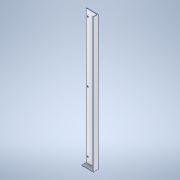
# Autodesk Inventor part: Guias de bandeja 1
Saved by Autodesk Inventor 2020 (Build 240168000, 168)
## iProperties
Created: 2020-05-08
Part Number: Guias de bandeja 1
Material: Aluminio 6061
Document SubType Name: Modeling
Designer: Pipi
Density: 2.7 g/cm^3
Appearance: Aluminio - Plano
Mass: 97.8928 g
Surface Area: 381.6 cm^2
Volume: 36.2566 cm^3
Author: Pipi
Autodesk Inventor part; units mm, degrees
ref_plane "YZ Plane" through (0, 0, 0) normal (1, 0, 0) x (0, 1, 0)
ref_plane "XZ Plane" through (0, 0, 0) normal (0, 1, 0) x (-1, 0, 0)
ref_plane "XY Plane" through (0, 0, 0) normal (0, 0, 1) x (1, 0, 0)
sketch "Boceto1" plane through (0, 0, 0) normal (0, 1, 0) x (-1, 0, 0)
  line L0 (25.8526, 17.8417) -> (25.8526, 15.8417)
  line L1 (25.8526, 15.8417) -> (-9.1474, 15.8417)
  line L2 (-9.1474, 15.8417) -> (-9.1474, 30.8417)
  line L3 (-9.1474, 30.8417) -> (-7.1474, 30.8417)
  line L4 (-7.1474, 30.8417) -> (-7.1474, 17.8417)
  line L5 (-7.1474, 17.8417) -> (25.8526, 17.8417)
  dimension "d0" = 2
  dimension "d1" = 35
  dimension "d2" = 15
  dimension "d3" = 2
  constraints: 12 end point, 5 perpendicular, 1 vertical
  measures "d0" distance of L0.start L0.end
  measures "d1" distance of L0.end L1.end
  measures "d2" distance of L1.end L2.end
  measures "d3" distance of L2.end L3.end
extrude "Extrusión1" add sketch "Boceto1" along normal blind 414
sketch "Boceto3" plane through (-25.8526, 0, 17.8417) normal (0, 0, 1) x (1, 0, 0)
  line L0 (35, 0) -> (0, 0) projected
  line L1 (35, 0) -> (5, 0)
  line L2 (5, 0) -> (5, 414)
  circle A0 centre (5, 20) radius 2
  circle A1 centre (5, 207) radius 2
  circle A2 centre (5, 394) radius 2
  line L3 (0, 414) -> (33, 414) projected
  dimension "d20" = 30
  dimension "d21" = 414
  dimension "d22" = 4
  dimension "d23" = 4
  dimension "d24" = 4
  dimension "d25" = 20
  dimension "d26" = 207
  dimension "d27" = 20
  constraints: 4 end point, 3 centre point, 3 point on line, 1 midpoint, 1 vertical
  measures "d20" distance of L0.start L1.end
  measures "d21" distance of L1.end L2.end
  measures "d22" diameter of A0
  measures "d23" diameter of A1
  measures "d24" diameter of A2
  measures "d25" distance of L1.end A0.centre
  measures "d26" distance from line of L0 A1.centre
  measures "d27" distance from line of L3 A2.centre
extrude "Extrusión2" cut sketch "Boceto3" against normal blind 10
sketch "Boceto5" plane through (0, 0, 0) normal (0, -1, 0) x (1, 0, 0)
  line L0 (-25.8526, 17.8417) -> (7.1474, 17.8417) projected
  line L1 (-25.8526, 17.8417) -> (-25.8526, 30.8417)
  line L2 (7.1474, 17.8417) -> (7.1474, 30.8417) projected
  line L3 (-25.8526, 30.8417) -> (7.1474, 30.8417)
  point P0 (0, 0)
  constraints: 4 end point, 1 perpendicular, 1 vertical
extrude "Extrusión4" add sketch "Boceto5" against normal blind 2
